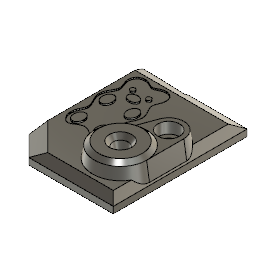
reverse_bowden (Autodesk Fusion 360 archive; units mm, degrees)
design "fs_cover" references "IR-sensor-01", "molex_sl_3pin"
Autodesk Fusion 360 part; units mm, degrees
sketch "base" plane through (0, 0, 0) normal (0, 0, 1) x (1, 0, 0)
  line L0 (0, 0) -> (28.1, 0)
  line L1 (28.1, 0) -> (28.1, 36)
  line L2 (28.1, 36) -> (0, 36)
  line L3 (0, 36) -> (0, 0)
  circle A0 centre (23, 20) radius 1.65
  circle A1 centre (20.05, 10) radius 1.3
  circle A2 centre (20.05, 10) radius 6.85
  line L4 (0, 5.374) -> (5.374, 0)
  circle A3 centre (23, 20) radius 2.9
  line L5 (26.9, 10) -> (26.9, 20)
  arc A4 (26.9, 20) -> (19.3352, 21.3339) centre (23, 20) ccw
  line L6 (14.05, 0) -> (14.05, 36) construction
  line L7 (19.3352, 21.3339) -> (17.5281, 16.3689)
  point P0 (20.05, 10)
  dimension "d4" = 3.3
  dimension "d7" = 2.6
  dimension "d11" = 2.95
  dimension "d78" = 10
  dimension "d85" = 20.05
  dimension "d94" = 8.05
  dimension "d139" = 10
  dimension "d142" = 45
  dimension "d160" = 5.8
  dimension "d163" = 26
  dimension "d260" = 3.8
  dimension "d300" = 0
  dimension "d301" = 0
  dimension "d302" = 0
  dimension "d303" = 0
  dimension "d340" = 0
  dimension "d341" = 0
  dimension "d342" = 0
  dimension "d343" = 0
  dimension "d390" = 110
  dimension "d391" = 1
  constraint horizontal L0
  constraint vertical L1
  constraint horizontal L2
  constraint vertical L3
  constraint coincident L0.start L3.end
  constraint coincident L3 L4.start
  constraint coincident L0 L4.end
  constraint coincident P0 A1.centre
  constraint concentric A0 A3
  constraint coincident A0.centre A3.centre
  constraint tangent L5 A4
  constraint vertical L5
  constraint tangent A2 L5
  constraint coincident A2 L5.start
  constraint coincident L0 L6.start
  constraint midpoint L2 L6.end
  constraint midpoint L0 L6.start
  constraint coincident A2 L7.end
  constraint tangent A4 L7
  measures "d4" diameter of A0
  measures "d7" diameter of A1
  measures "d11" horizontal distance of A0.centre P0
  measures "d78" vertical distance of L0.end P0
  measures "d85" horizontal distance of L0.start A1.centre
  measures "d94" horizontal distance of L0.end P0
  measures "d139" vertical distance of A0.centre P0
  measures "d142" angle of L3 L4
  measures "d160" diameter of A3
  measures "d163" distance of L2 P0
  measures "d260" distance of L0.start L4
  measures "d390" angle of L2 L7
  measures "d391" distance of A3 A4
extrude "Extrude1" add sketch "base" against normal blind 4 contours L0 L1 L2 L3 L4 | A2 | A2 L5 A4 L7 | A3
extrude "Extrude22" add sketch "base" along normal blind 4 contours A2
extrude "Extrude31" add sketch "base" along normal blind 3 contours A2 L5 A4 L7
draft "Draft3" angle 9 neutral plane through (0, 0, 4) pull (0, 0, 1) 4 faces at (26.9, 13.3333, 1) (24.6752, 23.5219, 2) (18.7328, 19.6789, 1) (26.866, 9.3182, 2.3333)
chamfer "Chamfer32" distance 1 angle 45 1 edges at (13.6636, 7.5229, 4)
chamfer "Chamfer4" distance 1.5 distance2 2.2 3 edges at (0, 20.687, 0) (28.1, 18, 0) (16.737, 0, 0) measured on face at (4.573, 18.4548, 0) measured on face at (4.573, 18.4548, 0) measured on face at (4.573, 18.4548, 0)
chamfer "Chamfer15" distance 3.6 distance2 2.2 2 edges at (14.05, 36, 0) (2.687, 2.687, 0) measured on face at (5.4116, 17.6551, 0) measured on face at (5.4116, 17.6551, 0)
chamfer "Chamfer23" distance 1 distance2 5 1 edges at (18.838, 10.4701, 4) measured on face at (24.3567, 10.3552, 4)
chamfer "Chamfer25" distance 1.3 distance2 0.7 1 edges at (17.9056, 9.1683, 4) measured on face at (20.5321, 7.8877, 3.3333)
chamfer "Chamfer24" distance 0.4 angle 45 1 edges at (21.4617, 19.4033, -4)
sketch "Sketch12" plane through (0, 0, -4) normal (0, 0, -1) x (1, 0, 0)
  line L0 (5.374, 0) -> (0, -5.374)
  line L1 (0, -5.374) -> (0, -36)
  line L2 (0, -36) -> (28.1, -36)
  line L3 (28.1, -36) -> (28.1, 0)
  line L4 (28.1, 0) -> (5.374, 0)
  line L5 (0, -36) -> (28.1, -36)
  circle A0 centre (23, -20) radius 2.05
  circle A1 centre (6.4, -19.362) radius 2
  line L6 (0.9896, -6.2838) -> (9.4572, -5.543)
  line L7 (9.4572, -5.543) -> (12.1219, -36)
  line L8 (3.5894, -36) -> (0.9896, -6.2838)
  line L9 (7.8556, -36) -> (5.2234, -5.9134) construction
  line L10 (2.8634, -27.702) -> (11.3311, -26.9611)
  line L11 (1.2075, -8.7743) -> (9.6751, -8.0334)
  line L12 (4.3577, -27.5712) -> (5.0951, -36)
  line L13 (5.0027, -34.9431) -> (10.4817, -34.4637)
  line L14 (10.6161, -36) -> (9.8368, -27.0919)
  line L15 (4.8894, -33.648) -> (6.2977, -34.8298)
  line L16 (12.0545, -35.2296) -> (3.2483, -36)
  line L17 (10.3684, -33.1687) -> (9.1867, -34.577)
  line L18 (14.0108, -5.85) -> (14.737, -14.15)
  line L19 (14.737, -14.15) -> (24.2, -14.15)
  line L20 (24.2, -14.15) -> (24.2, -5.85)
  line L21 (24.2, -5.85) -> (14.0108, -5.85)
  line L22 (18.55, -5.85) -> (18.55, -14.15)
  line L23 (21.55, -5.85) -> (21.55, -14.15)
  line L24 (18.55, -8.5) -> (21.55, -8.5)
  line L25 (18.55, -11.5) -> (21.55, -11.5)
  circle A2 centre (20.05, -10) radius 1.3
  circle A3 centre (20.05, -10) radius 1.5 construction
  dimension "d277" = 4
  dimension "d279" = 13.5
  dimension "d329" = 95
  dimension "d330" = 8
  dimension "d331" = 8.5
  dimension "d333" = 2.5
  dimension "d368" = 135
  dimension "d373" = 5.5
  dimension "d374" = 0.9
  dimension "d379" = 7.4
  dimension "d383" = 1.3
  dimension "d397" = 8.3
  dimension "d402" = 13.65
  dimension "d403" = 9.362
  dimension "d404" = 0.2
  dimension "d405" = 4.15
  dimension "d406" = 5.313
  dimension "d407" = 4.15
  constraint midpoint L6 L9.end
  constraint coincident L5 L9.start
  constraint coincident A1.centre L9
  constraint coincident L2 L8.start
  constraint coincident L2 L7.end
  constraint coincident L8 L10.start
  constraint coincident L7 L10.end
  constraint perpendicular L7 L10
  constraint perpendicular L6 L7
  constraint perpendicular L6 L8
  constraint perpendicular L6 L9
  constraint coincident L8 L11.start
  constraint coincident L7 L11.end
  constraint perpendicular L7 L11
  constraint coincident L10 L12.start
  constraint perpendicular L10 L12
  constraint perpendicular L9 L13
  constraint coincident L10 L14.end
  constraint perpendicular L10 L14
  constraint coincident L12 L15.start
  constraint coincident L2 L14.start
  constraint coincident L2 L12.end
  constraint perpendicular L14 L16
  constraint coincident L2 L16.end
  constraint coincident L7 L16.start
  constraint coincident L14 L13.end
  constraint coincident L12 L13.start
  constraint coincident L13 L15.end
  constraint symmetric L9 L15.start L17.start
  constraint symmetric L9 L15.end L17.end
  constraint horizontal L19
  constraint perpendicular L19 L20
  constraint perpendicular L20 L21
  constraint parallel L7 L18
  constraint coincident L21 L22.start
  constraint coincident L19 L22.end
  constraint coincident L21 L23.start
  constraint coincident L19 L23.end
  constraint parallel L22 L23
  constraint coincident L23 L24.end
  constraint coincident L22 L25.start
  constraint coincident L23 L25.end
  constraint perpendicular L23 L25
  constraint perpendicular L23 L24
  constraint perpendicular L21 L23
  constraint coincident L22 L24.start
  constraint concentric A2 A3
  constraint tangent L22 A3
  constraint tangent L23 A3
  constraint tangent L25 A3
  constraint tangent L24 A3
  measures "d277" diameter of A1
  measures "d279" distance of A1.centre L6
  measures "d329" angle of L2 L7
  measures "d330" distance of A1.centre L10
  measures "d331" distance of L7 L8
  measures "d333" distance of L6 L11
  measures "d368" angle of L13 L15
  measures "d373" distance of L12 L14
  measures "d374" distance of L13 L16
  measures "d379" distance of L10 L13
  measures "d383" distance of L13.start L15.end
  measures "d397" distance of L19 L21
  measures "d402" horizontal distance of A1.centre A2.centre
  measures "d403" vertical distance of A1.centre A2.centre
  measures "d404" distance of A2 A3
  measures "d405" distance of L20 A2.centre
  measures "d406" horizontal distance of L18.end A2.centre
  measures "d407" distance of L19 A2.centre
extrude "Extrude23" cut sketch "Sketch12" against normal blind 2.8 contours L7 L8 L10 L11 | A1
extrude "Extrude25" cut sketch "Sketch12" against normal blind 1.6 contours L6 L7 L8 L11
chamfer "Chamfer28" distance 1 distance2 1.4 2 edges at (10.5031, 17.4973, -1.2) (2.0354, 18.2381, -1.2) measured on face at (10.7791, 20.6519, -2.5333) measured on face at (2.3114, 21.3927, -2.5333)
chamfer "Chamfer29" distance 1 angle 45 1 edges at (7.0972, 27.3316, -1.2)
extrude "Extrude26" cut sketch "Sketch12" against normal blind 2 contours L18 L19 L21 L22 | L21 L22 L23 L24 | L19 L22 L23 L25 | L19 L20 L21 L23 | L22 L23 L24 L25 | A2
extrude "Extrude32" cut sketch "Sketch12" against normal blind 0.2 from surface at -2 contours L21 L22 L23 L24 | L19 L22 L23 L25
extrude "Extrude33" cut sketch "Sketch12" against normal blind 0.4 from surface at -2 contours L22 L23 L24 L25
chamfer "Chamfer33" distance 0.2 angle 45 1 edges at (18.838, 10.4701, -1.6)
chamfer "Chamfer30" distance 0.8 angle 45 2 edges at (22.875, 14.15, -2) (16.6435, 14.15, -2)
chamfer "Chamfer36" distance 1 angle 45 1 edges at (20.05, 14.15, -1.8)
chamfer "Chamfer34" distance 0.5 angle 45 2 edges at (16.2804, 5.85, -2) (22.875, 5.85, -2)
chamfer "Chamfer35" distance 0.7 angle 45 1 edges at (20.05, 5.85, -1.8)
extrude "Extrude27" cut sketch "Sketch12" against normal blind 1.8 contours L10 L12 L13 L14 L15 L17
extrude "Extrude28" cut sketch "Sketch12" against normal up to surface (4 mm away) contours L2 L5 L8 L16 | L2 L5 L7 L14 L16 | L2 L5 L8 L12 L16 | L2 L5 L12 L14 L16
extrude "Extrude29" cut sketch "Sketch12" against normal blind 0.4 contours L12 L13 L14 L16 | L12 L13 L15 | L13 L14 L17
extrude "Extrude30" cut sketch "Sketch12" against normal blind 0.2 from surface at -0.4 contours L12 L13 L15 | L13 L14 L17
chamfer "Chamfer31" distance 0.3 angle 45 11 edges at (10.1985, 31.2261, -4) (4.7194, 31.7054, -4) (10.5839, 27.0265, -4) (10.3941, 16.2521, -4) (3.6106, 27.6366, -4) (1.9265, 16.9929, -4) (5.2234, 5.9134, -4) (14.3739, 10, -4) (19.1054, 5.85, -4) (24.2, 10, -4) (19.4685, 14.15, -4)
chamfer "Chamfer37" distance 0.4 distance2 0.6 1 edges at (0.8271, 6.1474, -3.85) measured on face at (6.6172, 5.5907, -3.9)
sketch "logo" plane through (0, 0, 0) normal (0, 0, 1) x (-1, 0, 0)
  line L0 (-7.137, -30.9124) -> (-7.4972, -30.7692)
  line L1 (-7.4972, -30.7692) -> (-7.8497, -30.717)
  line L2 (-8.2018, -30.772) -> (-7.8497, -30.717)
  line L3 (-8.5609, -30.9181) -> (-8.2018, -30.772)
  line L4 (-8.9439, -31.121) -> (-8.5609, -30.9181)
  line L5 (-9.3684, -31.3355) -> (-8.9439, -31.121)
  line L6 (-9.8442, -31.515) -> (-9.3684, -31.3355)
  line L7 (-10.3649, -31.6212) -> (-9.8442, -31.515)
  line L8 (-10.9089, -31.6281) -> (-10.3649, -31.6212)
  line L9 (-11.4437, -31.5216) -> (-10.9089, -31.6281)
  line L10 (-11.9335, -31.2991) -> (-11.4437, -31.5216)
  line L11 (-12.3451, -30.9686) -> (-11.9335, -31.2991)
  line L12 (-12.6544, -30.5482) -> (-12.3451, -30.9686)
  line L13 (-12.8496, -30.0635) -> (-12.6544, -30.5482)
  line L14 (-12.9308, -29.544) -> (-12.8496, -30.0635)
  line L15 (-12.909, -29.0181) -> (-12.9308, -29.544)
  line L16 (-12.8044, -28.5094) -> (-12.909, -29.0181)
  line L17 (-12.6459, -28.0314) -> (-12.8044, -28.5094)
  line L18 (-12.4681, -27.5866) -> (-12.6459, -28.0314)
  line L19 (-12.3069, -27.169) -> (-12.4681, -27.5866)
  line L20 (-12.1948, -26.768) -> (-12.3069, -27.169)
  line L21 (-12.1559, -26.3719) -> (-12.1948, -26.768)
  line L22 (-12.2009, -25.9719) -> (-12.1559, -26.3719)
  line L23 (-12.3268, -25.5635) -> (-12.2009, -25.9719)
  line L24 (-12.5193, -25.1448) -> (-12.3268, -25.5635)
  line L25 (-12.756, -24.7153) -> (-12.5193, -25.1448)
  line L26 (-13.0095, -24.2743) -> (-12.756, -24.7153)
  line L27 (-13.2513, -23.8198) -> (-13.0095, -24.2743)
  line L28 (-13.454, -23.3491) -> (-13.2513, -23.8198)
  line L29 (-13.5938, -22.8596) -> (-13.454, -23.3491)
  line L30 (-13.6532, -22.3506) -> (-13.5938, -22.8596)
  line L31 (-13.6238, -21.8239) -> (-13.6532, -22.3506)
  line L32 (-13.5081, -21.2849) -> (-13.6238, -21.8239)
  line L33 (-13.3192, -20.7417) -> (-13.5081, -21.2849)
  line L34 (-13.0791, -20.2034) -> (-13.3192, -20.7417)
  line L35 (-12.8165, -19.6775) -> (-13.0791, -20.2034)
  line L36 (-12.5649, -19.1684) -> (-12.8165, -19.6775)
  line L37 (-12.361, -18.675) -> (-12.5649, -19.1684)
  line L38 (-12.2403, -18.1899) -> (-12.361, -18.675)
  line L39 (-12.2302, -17.7013) -> (-12.2403, -18.1899)
  line L40 (-12.3403, -17.1958) -> (-12.2302, -17.7013)
  line L41 (-12.5529, -16.6612) -> (-12.3403, -17.1958)
  line L42 (-12.8149, -16.0902) -> (-12.5529, -16.6612)
  line L43 (-13.0553, -15.4829) -> (-12.8149, -16.0902)
  line L44 (-13.222, -14.848) -> (-13.0553, -15.4829)
  line L45 (-13.285, -14.201) -> (-13.222, -14.848)
  line L46 (-13.2328, -13.5624) -> (-13.285, -14.201)
  line L47 (-13.0694, -12.9564) -> (-13.2328, -13.5624)
  line L48 (-12.8101, -12.4081) -> (-13.0694, -12.9564)
  line L49 (-12.4781, -11.9425) -> (-12.8101, -12.4081)
  line L50 (-12.101, -11.5815) -> (-12.4781, -11.9425)
  line L51 (-11.7053, -11.3416) -> (-12.101, -11.5815)
  line L52 (-11.3126, -11.2303) -> (-11.7053, -11.3416)
  line L53 (-10.9344, -11.2437) -> (-11.3126, -11.2303)
  line L54 (-10.5691, -11.3637) -> (-10.9344, -11.2437)
  line L55 (-10.2047, -11.5613) -> (-10.5691, -11.3637)
  line L56 (-9.827, -11.8002) -> (-10.2047, -11.5613)
  line L57 (-9.428, -12.0446) -> (-9.827, -11.8002)
  line L58 (-9.0137, -12.2633) -> (-9.428, -12.0446)
  line L59 (-8.6061, -12.4333) -> (-9.0137, -12.2633)
  line L60 (-8.2337, -12.5397) -> (-8.6061, -12.4333)
  line L61 (-7.9216, -12.5746) -> (-8.2337, -12.5397)
  line L62 (-7.9216, -12.5746) -> (-7.6098, -12.5373)
  line L63 (-7.6098, -12.5373) -> (-7.2383, -12.4278)
  line L64 (-7.2383, -12.4278) -> (-6.832, -12.2546)
  line L65 (-6.832, -12.2546) -> (-6.4196, -12.0328)
  line L66 (-6.4196, -12.0328) -> (-6.0224, -11.7852)
  line L67 (-6.0224, -11.7852) -> (-5.6466, -11.5431)
  line L68 (-5.6466, -11.5431) -> (-5.2838, -11.3428)
  line L69 (-5.2838, -11.3428) -> (-4.9194, -11.2198)
  line L70 (-4.9194, -11.2198) -> (-4.5414, -11.2035)
  line L71 (-4.5414, -11.2035) -> (-4.1478, -11.3116)
  line L72 (-4.1478, -11.3116) -> (-3.7502, -11.5484)
  line L73 (-3.7502, -11.5484) -> (-3.3703, -11.9064)
  line L74 (-3.3703, -11.9064) -> (-3.0347, -12.3693)
  line L75 (-3.0347, -12.3693) -> (-2.771, -12.9155)
  line L76 (-2.771, -12.9155) -> (-2.6028, -13.5203)
  line L77 (-2.6028, -13.5203) -> (-2.5456, -14.1583)
  line L78 (-2.5456, -14.1583) -> (-2.6034, -14.8059)
  line L79 (-2.6034, -14.8059) -> (-2.765, -15.4421)
  line L80 (-2.765, -15.4421) -> (-3.0006, -16.0513)
  line L81 (-3.0006, -16.0513) -> (-3.2581, -16.6244)
  line L82 (-3.2581, -16.6244) -> (-3.4665, -17.1606)
  line L83 (-3.4665, -17.1606) -> (-3.5725, -17.667)
  line L84 (-3.5725, -17.667) -> (-3.5586, -18.1556)
  line L85 (-3.5586, -18.1556) -> (-3.4341, -18.6396)
  line L86 (-3.4341, -18.6396) -> (-3.2262, -19.1314)
  line L87 (-3.2262, -19.1314) -> (-2.9706, -19.6385)
  line L88 (-2.9706, -19.6385) -> (-2.7039, -20.1623)
  line L89 (-2.7039, -20.1623) -> (-2.4595, -20.6987)
  line L90 (-2.4595, -20.6987) -> (-2.2662, -21.2403)
  line L91 (-2.2662, -21.2403) -> (-2.1463, -21.7784)
  line L92 (-2.1463, -21.7784) -> (-2.1128, -22.3049)
  line L93 (-2.1128, -22.3049) -> (-2.1681, -22.8144)
  line L94 (-2.1681, -22.8144) -> (-2.3039, -23.3049)
  line L95 (-2.3039, -23.3049) -> (-2.5029, -23.7772)
  line L96 (-2.5029, -23.7772) -> (-2.7412, -24.2336)
  line L97 (-2.7412, -24.2336) -> (-2.9912, -24.6766)
  line L98 (-2.9912, -24.6766) -> (-3.2243, -25.1079)
  line L99 (-3.2243, -25.1079) -> (-3.4135, -25.5282)
  line L100 (-3.4135, -25.5282) -> (-3.5363, -25.9375)
  line L101 (-3.5363, -25.9375) -> (-3.5781, -26.3378)
  line L102 (-3.5781, -26.3378) -> (-3.5361, -26.7336)
  line L103 (-3.5361, -26.7336) -> (-3.4208, -27.1338)
  line L104 (-3.4208, -27.1338) -> (-3.2562, -27.5501)
  line L105 (-3.2562, -27.5501) -> (-3.0748, -27.9934)
  line L106 (-3.0748, -27.9934) -> (-2.9126, -28.4701)
  line L107 (-2.9126, -28.4701) -> (-2.8041, -28.9781)
  line L108 (-2.8041, -28.9781) -> (-2.7781, -29.5037)
  line L109 (-2.7781, -29.5037) -> (-2.8551, -30.0239)
  line L110 (-2.8551, -30.0239) -> (-3.0466, -30.5101)
  line L111 (-3.0466, -30.5101) -> (-3.3524, -30.9329)
  line L112 (-3.3524, -30.9329) -> (-3.7614, -31.2667)
  line L113 (-3.7614, -31.2667) -> (-4.2494, -31.4931)
  line L114 (-4.2494, -31.4931) -> (-4.7834, -31.6038)
  line L115 (-4.7834, -31.6038) -> (-5.3274, -31.6012)
  line L116 (-5.3274, -31.6012) -> (-5.8491, -31.4991)
  line L117 (-5.8491, -31.4991) -> (-6.3262, -31.3234)
  line L118 (-6.3262, -31.3234) -> (-6.7524, -31.1124)
  line L119 (-6.7524, -31.1124) -> (-7.137, -30.9124)
  spline S0 degree 3 poles (-10.0133, -26.9939) (-10.3655, -26.9939) (-10.6511, -27.2794) (-10.6511, -27.6317) knots 0 0 0 0 1 1 1 1
  spline S1 degree 3 poles (-10.6511, -27.6317) (-10.6511, -27.9839) (-10.3655, -28.2693) (-10.0133, -28.2693) knots 0 0 0 0 1 1 1 1
  spline S2 degree 3 poles (-9.3756, -27.6317) (-9.3756, -27.2794) (-9.6612, -26.9939) (-10.0133, -26.9939) knots 0 0 0 0 1 1 1 1
  spline S3 degree 3 poles (-10.0133, -28.2693) (-9.6612, -28.2693) (-9.3756, -27.9839) (-9.3756, -27.6317) knots 0 0 0 0 1 1 1 1
  spline S4 degree 3 poles (-5.0729, -27.6146) (-5.0729, -27.2624) (-5.3584, -26.9768) (-5.7107, -26.9768) knots 0 0 0 0 1 1 1 1
  spline S5 degree 3 poles (-5.7107, -26.9768) (-6.0629, -26.9768) (-6.3484, -27.2624) (-6.3484, -27.6146) knots 0 0 0 0 1 1 1 1
  spline S6 degree 3 poles (-5.7107, -28.2523) (-5.3585, -28.2523) (-5.0729, -27.9668) (-5.0729, -27.6146) knots 0 0 0 0 1 1 1 1
  spline S7 degree 3 poles (-6.3484, -27.6146) (-6.3484, -27.9668) (-6.0629, -28.2523) (-5.7107, -28.2523) knots 0 0 0 0 1 1 1 1
  spline S8 degree 3 poles (-7.8742, -24.5109) (-8.7358, -24.5144) (-9.4322, -25.0264) (-9.4297, -25.6545) knots 0 0 0 0 1 1 1 1
  spline S9 degree 3 poles (-9.4297, -25.6545) (-9.4272, -26.2827) (-8.7268, -26.7891) (-7.8653, -26.7857) knots 0 0 0 0 1 1 1 1
  spline S10 degree 3 poles (-6.3098, -25.6422) (-6.3123, -25.014) (-7.0127, -24.5076) (-7.8742, -24.5109) knots 0 0 0 0 1 1 1 1
  spline S11 degree 3 poles (-7.8653, -26.7857) (-7.0037, -26.7823) (-6.3073, -26.2704) (-6.3098, -25.6422) knots 0 0 0 0 1 1 1 1
  spline S12 degree 3 poles (-4.5451, -20.1948) (-5.3017, -20.1948) (-5.915, -20.9998) (-5.915, -21.9928) knots 0 0 0 0 1 1 1 1
  spline S13 degree 3 poles (-5.915, -21.9928) (-5.915, -22.9858) (-5.3017, -23.7909) (-4.5451, -23.7909) knots 0 0 0 0 1 1 1 1
  spline S14 degree 3 poles (-3.1751, -21.9928) (-3.1751, -20.9998) (-3.7885, -20.1948) (-4.5451, -20.1948) knots 0 0 0 0 1 1 1 1
  spline S15 degree 3 poles (-4.5451, -23.7909) (-3.7885, -23.7909) (-3.1751, -22.9859) (-3.1751, -21.9928) knots 0 0 0 0 1 1 1 1
  spline S16 degree 3 poles (-11.2376, -20.2213) (-11.9942, -20.2273) (-12.6011, -21.0372) (-12.5933, -22.0301) knots 0 0 0 0 1 1 1 1
  spline S17 degree 3 poles (-12.5933, -22.0301) (-12.5854, -23.0231) (-11.9657, -23.8232) (-11.2091, -23.8172) knots 0 0 0 0 1 1 1 1
  spline S18 degree 3 poles (-9.8535, -22.0085) (-9.8614, -21.0154) (-10.4811, -20.2154) (-11.2376, -20.2213) knots 0 0 0 0 1 1 1 1
  spline S19 degree 3 poles (-11.2091, -23.8172) (-10.4525, -23.8113) (-9.8456, -23.0014) (-9.8535, -22.0085) knots 0 0 0 0 1 1 1 1
  spline S20 degree 3 poles (-4.8393, -15.8282) (-4.0827, -15.8282) (-3.4694, -15.0232) (-3.4694, -14.0302) knots 0 0 0 0 1 1 1 1
  spline S21 degree 3 poles (-3.4694, -14.0302) (-3.4694, -13.0371) (-4.0828, -12.2322) (-4.8393, -12.2322) knots 0 0 0 0 1 1 1 1
  spline S22 degree 3 poles (-6.2092, -14.0302) (-6.2092, -15.0232) (-5.5959, -15.8282) (-4.8393, -15.8282) knots 0 0 0 0 1 1 1 1
  spline S23 degree 3 poles (-4.8393, -12.2322) (-5.5958, -12.2322) (-6.2092, -13.0371) (-6.2092, -14.0302) knots 0 0 0 0 1 1 1 1
  spline S24 degree 3 poles (-10.978, -15.8525) (-10.2215, -15.8465) (-9.6145, -15.0366) (-9.6224, -14.0436) knots 0 0 0 0 1 1 1 1
  spline S25 degree 3 poles (-9.6224, -14.0436) (-9.6303, -13.0507) (-10.25, -12.2506) (-11.0065, -12.2566) knots 0 0 0 0 1 1 1 1
  spline S26 degree 3 poles (-12.3622, -14.0654) (-12.3544, -15.0584) (-11.7346, -15.8585) (-10.978, -15.8525) knots 0 0 0 0 1 1 1 1
  spline S27 degree 3 poles (-11.0065, -12.2566) (-11.7631, -12.2626) (-12.3701, -13.0724) (-12.3622, -14.0654) knots 0 0 0 0 1 1 1 1
extrude "Extrude9" cut sketch "logo" against normal blind 0.4
equation "m3_holes = 3.3 mm"
equation "d4 = m3_holes"
equation "m3_head = 6 mm"
equation "layer_height = 0.2 mm"
equation "d64 = -layer_height * 2"
equation "center_extruder_to_motor_screw = 11.25 mm"
equation "d160 = m3_head - 0.2 mm"
equation "extrusion_width = 0.45 mm"
equation "num_perimeters = 4"
equation "num_top_bottoms = 5"
equation "perimeters_thickness = num_perimeters * ( extrusion_width - 0.05 mm )"
equation "top_bottom_thickness = layer_height * num_top_bottoms"
equation "light_leak_clearance = 0.3 mm"
equation "d265 = ( ( 4.5 - 2.5 ) / 2 ) * 1 mm"
equation "d381 = -layer_height * 2"
equation "d385 = -layer_height"
equation "d397 = d407 * 2"
equation "d405 = 4 mm + 0.15 mm"
equation "d406 = 5.163 mm + 0.15 mm"
equation "d407 = 4 mm + 0.15 mm"
equation "d408 = -layer_height"
equation "d412 = -layer_height * 2"
equation "d416 = 0.5 mm + layer_height"
equation "d417 = 0.8 mm + layer_height"
